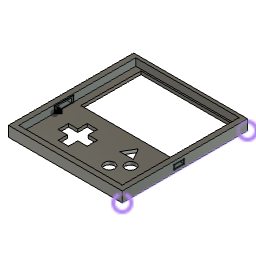
Enclosure BMO v13 (Autodesk Fusion 360 design; units mm, degrees)
Autodesk Fusion 360 part; units mm, degrees
sketch "Sketch1" plane through (0, 0, 0) normal (0, 0, 1) x (1, 0, 0)
  line L0 (-50.4372, 47.8193) -> (49.5628, 47.8193)
  line L1 (49.5628, 47.8193) -> (49.5628, -63.1807)
  line L2 (49.5628, -63.1807) -> (-50.4372, -63.1807)
  line L3 (-50.4372, -63.1807) -> (-50.4372, 47.8193)
  line L4 (-18.6372, -27.5802) -> (-23.0372, -27.5802)
  line L5 (-23.0372, -27.5802) -> (-23.0372, -24.2802)
  line L6 (-23.0372, -24.2802) -> (-18.6372, -24.2802)
  line L7 (-18.6372, -24.2802) -> (-18.6372, -27.5802)
  line L8 (17.6628, -24.0807) -> (22.0628, -24.0807)
  line L9 (22.0628, -24.0807) -> (22.0628, -27.3807)
  line L10 (22.0628, -27.3807) -> (17.6628, -27.3807)
  line L11 (17.6628, -27.3807) -> (17.6628, -24.0807)
  line L12 (17.8378, -44.4057) -> (22.2378, -44.4057)
  line L13 (22.2378, -44.4057) -> (22.2378, -47.7057)
  line L14 (22.2378, -47.7057) -> (17.8378, -47.7057)
  line L15 (17.8378, -47.7057) -> (17.8378, -44.4057)
  line L16 (27.9628, -34.1807) -> (32.3628, -34.1807)
  line L17 (32.3628, -34.1807) -> (32.3628, -37.4807)
  line L18 (32.3628, -37.4807) -> (27.9628, -37.4807)
  line L19 (27.9628, -37.4807) -> (27.9628, -34.1807)
  line L20 (-33.0372, -34.1807) -> (-28.6372, -34.1807)
  line L21 (-28.6372, -34.1807) -> (-28.6372, -37.4807)
  line L22 (-28.6372, -37.4807) -> (-33.0372, -37.4807)
  line L23 (-33.0372, -37.4807) -> (-33.0372, -34.1807)
  line L24 (-13.0372, -34.1807) -> (-8.6372, -34.1807)
  line L25 (-8.6372, -34.1807) -> (-8.6372, -37.4807)
  line L26 (-8.6372, -37.4807) -> (-13.0372, -37.4807)
  line L27 (-13.0372, -37.4807) -> (-13.0372, -34.1807)
  line L28 (-23.4439, -44.4057) -> (-19.0439, -44.4057)
  line L29 (-19.0439, -44.4057) -> (-19.0439, -47.7057)
  line L30 (-19.0439, -47.7057) -> (-23.4439, -47.7057)
  line L31 (-23.4439, -47.7057) -> (-23.4439, -44.4057)
  dimension "d1" = 100
  dimension "d2" = 111
  dimension "d3" = 4.4
  dimension "d4" = 3.3
  dimension "d5" = 4.4
  dimension "d6" = 3.3
  dimension "d7" = 4.4
  dimension "d8" = 3.3
  dimension "d9" = 4.4
  dimension "d10" = 3.3
  dimension "d11" = 4.4
  dimension "d12" = 3.3
  dimension "d13" = 4.4
  dimension "d14" = 3.3
  dimension "d15" = 4.4
  dimension "d16" = 3.3
  dimension "d17" = 17.4
  dimension "d21" = 25.7
  dimension "d22" = 25.7
  dimension "d23" = 15.475
  dimension "d24" = 15.475
  dimension "d25" = 25.7
  dimension "d26" = 27.5
  dimension "d27" = 17.2
  dimension "d28" = 15.6
  dimension "d29" = 8.656
  dimension "d30" = 8.656
  dimension "d31" = 8.656
  dimension "d32" = 35.8
  dimension "d33" = 27.325
  constraint horizontal L0
  constraint vertical L1
  constraint horizontal L2
  constraint vertical L3
  constraint horizontal L4
  constraint vertical L5
  constraint horizontal L6
  constraint vertical L7
  constraint horizontal L8
  constraint vertical L9
  constraint horizontal L10
  constraint vertical L11
  constraint horizontal L12
  constraint vertical L13
  constraint horizontal L14
  constraint vertical L15
  constraint horizontal L16
  constraint vertical L17
  constraint horizontal L18
  constraint vertical L19
  constraint horizontal L20
  constraint vertical L21
  constraint horizontal L22
  constraint vertical L23
  constraint horizontal L24
  constraint vertical L25
  constraint horizontal L26
  constraint vertical L27
  constraint horizontal L28
  constraint vertical L29
  constraint horizontal L30
  constraint vertical L31
  measures "d1" distance of L0.start L0.end
  measures "d2" distance of L0.end L1.end
  measures "d3" distance of L4.start L4.end
  measures "d4" distance of L4.end L5.end
  measures "d5" distance of L28.start L28.end
  measures "d6" distance of L28.end L29.end
  measures "d7" distance of L24.start L24.end
  measures "d8" distance of L24.end L25.end
  measures "d9" distance of L20.start L20.end
  measures "d10" distance of L20.end L21.end
  measures "d11" distance of L8.start L8.end
  measures "d12" distance of L8.end L9.end
  measures "d13" distance of L16.start L16.end
  measures "d14" distance of L16.end L17.end
  measures "d15" distance of L12.start L12.end
  measures "d16" distance of L12.start L14.end
  measures "d17" distance of L3 L23
  measures "d21" distance of L2 L22
  measures "d22" distance of L2 L26
  measures "d23" distance of L2 L30
  measures "d24" distance of L2 L14
  measures "d25" distance of L2 L18
  measures "d26" distance of L1 L9
  measures "d27" distance of L1 L17
  measures "d28" distance of L21 L27
  measures "d29" distance of L4.end L20.end
  measures "d30" distance of L4.start L24.start
  measures "d31" distance of L21.end L28.start
  measures "d32" distance of L2 L10
  measures "d33" distance of L1 L13
sketch "top enclosure" plane through (0, 0, 0) normal (0, 0, 1) x (1, 0, 0)
  circle A0 centre (30.5628, -36.1807) radius 5.15
  line L0 (20.0628, -18.1807) -> (13.3583, -29.4363)
  line L1 (13.3583, -29.4363) -> (26.3583, -29.4363)
  line L2 (26.3583, -29.4363) -> (20.0628, -18.1807)
  circle A1 centre (20.0628, -46.1807) radius 5.15
  line L3 (-25.9372, -21.6807) -> (-15.9372, -21.6807)
  line L4 (-15.9372, -21.6807) -> (-15.9372, -30.6807)
  line L5 (-15.9372, -30.6807) -> (-6.9372, -30.6807)
  line L6 (-6.9372, -30.6807) -> (-6.9372, -40.6807)
  line L7 (-6.9372, -40.6807) -> (-15.9372, -40.6807)
  line L8 (-15.9372, -40.6807) -> (-15.9372, -49.6807)
  line L9 (-15.9372, -49.6807) -> (-25.9372, -49.6807)
  line L10 (-25.9372, -49.6807) -> (-25.9372, -40.6807)
  line L11 (-25.9372, -40.6807) -> (-34.9372, -40.6807)
  line L12 (-34.9372, -40.6807) -> (-34.9372, -30.6807)
  line L13 (-34.9372, -30.6807) -> (-25.9372, -30.6807)
  line L14 (-25.9372, -30.6807) -> (-25.9372, -21.6807)
  line L15 (-55.4372, 52.8193) -> (54.5628, 52.8193)
  line L16 (54.5628, 52.8193) -> (54.5628, -68.1807)
  line L17 (54.5628, -68.1807) -> (-55.4372, -68.1807)
  line L18 (-55.4372, -68.1807) -> (-55.4372, 52.8193)
  line L19 (-50.4372, -63.1807) -> (-50.4372, 47.8193)
  line L20 (49.5628, -63.1807) -> (-50.4372, -63.1807)
  line L21 (49.5628, 47.8193) -> (49.5628, -63.1807)
  line L22 (-50.4372, 47.8193) -> (49.5628, 47.8193)
  line L23 (-43.9372, 48.3193) -> (45.0628, 48.3193)
  line L24 (45.0628, 48.3193) -> (45.0628, -9.6807)
  line L25 (45.0628, -9.6807) -> (-43.9372, -9.6807)
  line L26 (-43.9372, -9.6807) -> (-43.9372, 48.3193)
  line L27 (-23.0372, -24.2802) -> (-18.6372, -24.2802)
  line L28 (-50.4372, -63.1807) -> (49.5628, -63.1807)
  line L29 (49.5628, -63.1807) -> (49.5628, 49.8193)
  line L30 (49.5628, 49.8193) -> (-50.4372, 49.8193)
  line L31 (-50.4372, 49.8193) -> (-50.4372, -63.1807)
  line L32 (44.9628, -13.6807) -> (49.5628, -13.6807)
  line L33 (49.5628, -13.6807) -> (49.5628, -23.1807)
  line L34 (49.5628, -23.1807) -> (44.9628, -23.1807)
  line L35 (44.9628, -23.1807) -> (44.9628, -13.6807)
  line L36 (-50.4372, -5.1807) -> (-36.8011, -5.1807)
  line L37 (-36.8011, -5.1807) -> (-36.8011, -27.1807)
  line L38 (-36.8011, -27.1807) -> (-50.4372, -27.1807)
  line L39 (-50.4372, -27.1807) -> (-50.4372, -5.1807)
  dimension "d34" = 60
  dimension "d35" = 10.3
  dimension "d36" = 10.3
  dimension "d37" = 10
  dimension "d38" = 10
  dimension "d39" = 10
  dimension "d40" = 10
  dimension "d41" = 9
  dimension "d42" = 9
  dimension "d43" = 9
  dimension "d44" = 9
  dimension "d45" = 9
  dimension "d46" = 9
  dimension "d47" = 13
  dimension "d49" = 11.2555
  dimension "d50" = 5
  dimension "d51" = 5
  dimension "d52" = 5
  dimension "d53" = 5
  dimension "d54" = 89
  dimension "d55" = 58
  dimension "d56" = 6.5
  dimension "d59" = 14.5995
  dimension "d60" = 45
  dimension "d61" = 27
  dimension "d62" = 17
  dimension "d63" = 13.5
  dimension "d64" = 15.5
  dimension "d65" = 19
  dimension "d66" = 29.5
  dimension "d68" = 113
  dimension "d69" = 100
  dimension "d72" = 40
  dimension "d73" = 9.5
  dimension "d74" = 4.6
  dimension "d75" = 36
  dimension "d77" = 22
  constraint horizontal L1
  constraint horizontal L3
  constraint perpendicular L3 L4
  constraint perpendicular L4 L5
  constraint perpendicular L5 L6
  constraint perpendicular L6 L7
  constraint perpendicular L7 L8
  constraint perpendicular L8 L9
  constraint perpendicular L9 L10
  constraint perpendicular L10 L11
  constraint perpendicular L11 L12
  constraint perpendicular L12 L13
  constraint perpendicular L3 L14
  constraint horizontal L15
  constraint vertical L16
  constraint horizontal L17
  constraint vertical L18
  constraint horizontal L23
  constraint vertical L24
  constraint horizontal L25
  constraint vertical L26
  constraint horizontal L28
  constraint vertical L29
  constraint horizontal L30
  constraint vertical L31
  constraint coincident L19.start L20.end
  constraint horizontal L32
  constraint vertical L33
  constraint horizontal L34
  constraint vertical L35
  constraint coincident L21 L33.end
  constraint horizontal L36
  constraint vertical L37
  constraint horizontal L38
  constraint vertical L39
  constraint coincident L19 L36.start
  measures "d34" angle of L0 L2
  measures "d35" diameter of A1
  measures "d36" diameter of A0
  measures "d37" distance of L3.start L3.end
  measures "d38" distance of L8.end L9.end
  measures "d39" distance of L5.end L6.end
  measures "d40" distance of L11.end L12.end
  measures "d41" distance of L3.start L13.end
  measures "d42" distance of L3.end L4.end
  measures "d43" distance of L4.end L5.end
  measures "d44" distance of L6.end L7.end
  measures "d45" distance of L9.end L10.end
  measures "d46" distance of L12.end L13.end
  measures "d47" distance of L0.end L1.end
  measures "d49" distance of L0.start L1
  measures "d50" distance of L18 L19
  measures "d51" distance of L17 L20
  measures "d52" distance of L16 L21
  measures "d53" distance of L15 L22
  measures "d54" distance of L23.start L23.end
  measures "d55" distance of L23.end L24.end
  measures "d56" distance of L19 L26
  measures "d59" distance of L25 L27
  measures "d60" distance of L0.start L20
  measures "d61" distance of A0.centre L20
  measures "d62" distance of A1.centre L20
  measures "d63" distance of L9 L20
  measures "d64" distance of L12 L19
  measures "d65" distance of A0.centre L21
  measures "d66" distance of L0.start L21
  measures "d68" distance of L19.start L30.end
  measures "d69" distance of L19.start L20.start
  measures "d72" distance of L20 L34
  measures "d73" distance of L32 L34
  measures "d74" distance of L33 L35
  measures "d75" distance of L28 L38
  measures "d77" distance of L36.end L37.end
extrude "Extrude6" add sketch "top enclosure" along normal blind 10 contours L15 L16 L17 L18
extrude "Extrude7" add sketch "top enclosure" along normal blind 3 contours L19 L20 L21 L22 L24 L25 L28 L29 L31 L32 L34 L35 L37 L38 | L19 L25 L26 L31 L36 L37 L38 L39 | L19 L22 L26 L31 L36 | L21 L29 L32 L33 L34 L35 | L22 L23 L24 L26 L29 L30 L31
sketch "Sketch3" plane through (54.5628, 0, 0) normal (1, 0, 0) x (0, 1, 0)
  line L0 (-68.1807, 0) -> (52.8193, 0)
  line L1 (52.8193, 0) -> (52.8193, 10)
  line L2 (52.8193, 10) -> (-68.1807, 10)
  line L3 (-68.1807, 10) -> (-68.1807, 0)
  line L4 (-18.1807, 7) -> (-8.6807, 7)
  line L5 (-8.6807, 7) -> (-8.6807, 3)
  line L6 (-8.6807, 3) -> (-18.1807, 3)
  line L7 (-18.1807, 3) -> (-18.1807, 7)
  line L8 (52.8193, 0) -> (-68.1807, 0)
  dimension "d91" = 50
  dimension "d92" = 3
  dimension "d93" = 9.5
  dimension "d94" = 4
  constraint horizontal L4
  constraint vertical L5
  constraint horizontal L6
  constraint vertical L7
  measures "d91" distance of L3 L7
  measures "d92" distance of L6 L8
  measures "d93" distance of L4.start L4.end
  measures "d94" distance of L4.end L5.end
extrude "Extrude8" cut sketch "Sketch3" against normal blind 10 contours L4 L5 L6 L7
sketch "Sketch4" plane through (49.5628, 0, 0) normal (-1, 0, 0) x (0, -1, 0)
  line L0 (8.6807, 3) -> (8.6807, 7)
  line L1 (8.6807, 7) -> (18.1807, 7)
  line L2 (18.1807, 7) -> (18.1807, 3)
  line L3 (18.1807, 3) -> (63.1807, 3)
  line L4 (63.1807, 3) -> (63.1807, 10)
  line L5 (63.1807, 10) -> (-49.8193, 10)
  line L6 (-49.8193, 10) -> (-49.8193, 3)
  line L7 (-49.8193, 3) -> (8.6807, 3)
  line L8 (7.4307, 3) -> (19.4307, 3)
  line L9 (19.4307, 3) -> (19.4307, 8.6)
  line L10 (19.4307, 8.6) -> (7.4307, 8.6)
  line L11 (7.4307, 8.6) -> (7.4307, 3)
  line L12 (8.6807, 7) -> (8.6807, 3)
  dimension "d97" = 12
  dimension "d98" = 5.6
  dimension "d99" = 1.25
  constraint horizontal L8
  constraint vertical L9
  constraint horizontal L10
  constraint vertical L11
  constraint coincident L7 L8.start
  measures "d97" distance of L9.end L10.end
  measures "d98" distance of L8.end L9.end
  measures "d99" distance of L11 L12
extrude "Extrude9" cut sketch "Sketch4" against normal blind 2 contours L0 L1 L2 L3 L7 L8 L9 L10 L11 L12
sketch "Sketch5" plane through (-55.4372, 0, 0) normal (-1, 0, 0) x (0, -1, 0)
  line L0 (-52.8193, 0) -> (68.1807, 0)
  line L1 (68.1807, 0) -> (68.1807, 10)
  line L2 (68.1807, 10) -> (-52.8193, 10)
  line L3 (-52.8193, 10) -> (-52.8193, 0)
  line L4 (12.1807, 7.5) -> (27.1807, 7.5)
  line L5 (27.1807, 7.5) -> (27.1807, 3)
  line L6 (27.1807, 3) -> (12.1807, 3)
  line L7 (12.1807, 3) -> (12.1807, 7.5)
  dimension "d102" = 41
  dimension "d103" = 15
  dimension "d104" = 3
  dimension "d105" = 4.5
  constraint horizontal L4
  constraint vertical L5
  constraint horizontal L6
  constraint vertical L7
  measures "d102" distance of L1 L5
  measures "d103" distance of L4.start L4.end
  measures "d104" distance of L0 L6
  measures "d105" distance of L4.end L5.end
extrude "Extrude10" cut sketch "Sketch5" against normal blind 9 contours L4 L5 L6 L7
sketch "Sketch6" plane through (-50.4372, 0, 0) normal (1, 0, 0) x (0, 1, 0)
  line L0 (-27.1807, 3) -> (-27.1807, 7.5)
  line L1 (-27.1807, 7.5) -> (-12.1807, 7.5)
  line L2 (-12.1807, 7.5) -> (-12.1807, 3)
  line L3 (-12.1807, 3) -> (49.8193, 3)
  line L4 (49.8193, 3) -> (49.8193, 10)
  line L5 (49.8193, 10) -> (-63.1807, 10)
  line L6 (-63.1807, 10) -> (-63.1807, 3)
  line L7 (-63.1807, 3) -> (-27.1807, 3)
  line L8 (-28.6807, 3) -> (-10.6807, 3)
  line L9 (-10.6807, 3) -> (-10.6807, 9)
  line L10 (-10.6807, 9) -> (-28.6807, 9)
  line L11 (-28.6807, 9) -> (-28.6807, 3)
  dimension "d108" = 1.5
  dimension "d111" = 18
  dimension "d112" = 6
  constraint horizontal L8
  constraint vertical L9
  constraint horizontal L10
  constraint vertical L11
  constraint coincident L7 L8.start
  measures "d108" distance of L2 L9
  measures "d111" distance of L9.end L10.end
  measures "d112" distance of L8.start L10.end
extrude "Extrude11" [suppressed]
named bodies: "Top Part"
